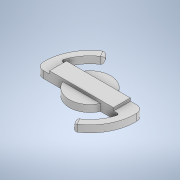
# Autodesk Inventor part: Servo_Kupplung
Saved by Autodesk Inventor 2020 (Build 240168000, 168)
## iProperties
Created: 2020-09-04
Part Number: Servo_Kupplung
Material: Generisch
Document SubType Name: Modeling
Designer: sp
Density: 1 g/cm^3
Appearance: Vorgabe
Author: sp
## iProperties of the stored document _3D-Druck.ipt
Created: 2020-09-04
Part Number: _3D-Druck
Material: Generisch
Document SubType Name: Modeling
Designer: sp
Density: 1 g/cm^3
Appearance: Vorgabe
Author: sp
Autodesk Inventor part; units mm, degrees
ref_plane "YZ Plane" through (0, 0, 0) normal (1, 0, 0) x (0, 1, 0)
ref_plane "XZ Plane" through (0, 0, 0) normal (0, 1, 0) x (-1, 0, 0)
ref_plane "XY Plane" through (0, 0, 0) normal (0, 0, 1) x (1, 0, 0)
sketch "Skizze1" plane through (0, 0, 0) normal (0, 1, 0) x (-1, 0, 0)
  circle A0 centre (0, 0) radius 24.25
  circle A1 centre (0, 0) radius 20.75
  circle A2 centre (0, 0) radius 3.5
  line L0 (45.7225, 0) -> (-63.662, 0) construction
  line L1 (0, 78.2374) -> (0, -78.2374) construction
  circle A3 centre (15, 0) radius 2
  circle A4 centre (-15, 0) radius 2
  line L2 (0, 3.5) -> (15.1977, 1.9902)
  line L3 (15.1977, -1.9902) -> (0, -3.5)
  line L4 (-14.8023, -1.9902) -> (0, -3.5)
  line L5 (0, 3.5) -> (-15.1977, 1.9902)
  circle A5 centre (0, 0) radius 11
  line L6 (10.0387, 4.4973) -> (20.2568, 4.4973)
  line L7 (-10.0387, 4.4973) -> (-20.2568, 4.4973)
  line L8 (10.0387, -4.4973) -> (20.2568, -4.4973)
  line L9 (20.2568, 4.4973) -> (23.8293, 4.4973)
  line L10 (-20.2568, 4.4973) -> (-29, 4.4973)
  line L11 (-10.0387, -4.4973) -> (-23.8293, -4.4973)
  line L12 (12.125, -21.0011) -> (-12.125, 21.0011)
  point P0 (-0.6886, 3.4316)
  point P1 (0.6886, 3.4316)
  point P2 (0.6886, -3.4316)
  point P3 (-0.7066, -3.4279)
  point P4 (-10.375, 17.97)
  point P5 (10.375, -17.97)
  dimension "d0" = 48.5
  dimension "d1" = 41.5
  dimension "d2" = 7
  dimension "d3" = 4
  dimension "d4" = 4
  dimension "d5" = 15
  dimension "d6" = 22
  dimension "d10" = 120
  constraints: 26 end point, 17 point on circle, 10 point on line, 6 centre point, 4 coincident, 3 horizontal, 3 midpoint, 1 parallel, 1 symmetric about line, 1 tangent, 1 vertical
  measures "d0" diameter of A0
  measures "d1" diameter of A1
  measures "d2" diameter of A2
  measures "d3" diameter of A3
  measures "d4" diameter of A4
  measures "d5" distance of point (0, 0) A3.centre
  measures "d6" diameter of A5
  measures "d10" angle of L0 L12
extrude "Extrusion1" add sketch "Skizze1" along normal blind 3.7 contours A0 L12 A1 L9 | L12 A1 L10 A0 | A1 L8 A5 L3 A3 L2 L6 | A0 L10 A1 L11 | A5 L2 A2 L5 L12 | A1 L7 A5 L5 A4 L4 L11 | L12 L3 A5 | A5 L4 A2 L3 L12 | L12 L5 A5 picked at (14.067, -18.158)
fillet "Rundung1" radius 4 2 edges at (-23.8293, 1.85, 4.4973) (23.8293, 1.85, -4.4973)
sketch "Skizze2" plane through (0, 3.7, 0) normal (0, 1, 0) x (1, 0, 0)
  line L0 (-10.0387, 4.4973) -> (-20.2568, 4.4973) projected
  line L1 (10.0387, -4.4973) -> (20.2568, -4.4973) projected
  line L2 (-17, 4.4973) -> (16.9902, 4.4973)
  line L3 (16.9902, 4.4973) -> (16.9902, -4.4973)
  line L4 (16.9902, -4.4973) -> (-17, -4.4973)
  line L5 (-17, -4.4973) -> (-17, 4.4973)
  arc A0 (15.1977, -1.9902) -> (14.8023, 1.9902) centre (15, 0) ccw projected
  arc A1 (-15.1977, 1.9902) -> (-15.1977, -1.9902) centre (-15, 0) ccw projected
  point P0 (0, 0)
  point P1 (10.0387, -4.4973)
  point P2 (-10.0387, 4.4973)
  point P3 (16.9902, 0.1977)
  point P4 (-17, 0)
  constraints: 8 end point, 3 point on line, 2 parallel, 2 point on circle, 1 horizontal, 1 midpoint, 1 perpendicular
extrude "Extrusion2" add sketch "Skizze2" along normal blind 1.5 contours L2 L3 L1 L4 L5 L0
fillet "Rundung2" radius 1 2 edges at (20.2568, 1.85, 4.4973) (-20.2568, 1.85, -4.4973)
fillet "Rundung3" radius 1.5 4 edges at (10.375, 1.85, 17.97) (11.25, 3.7, 19.4856) (12.125, 1.85, 21.0011) (11.25, 0, 19.4856)
fillet "Rundung4" radius 1.5 4 edges at (-11.25, 3.7, -19.4856) (-12.125, 1.85, -21.0011) (-11.25, 0, -19.4856) (-10.375, 1.85, -17.97)
